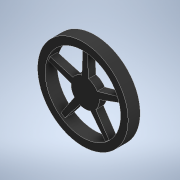
# Autodesk Inventor part: FS90R-W
Saved by Autodesk Inventor 2022 (Build 260153000, 153)
## iProperties
Created: 2024-05-30
Part Number: FS90R-W
Material: 一般
Document SubType Name: Modeling
Designer: yamashita1
Density: 1 g/cm^3
Appearance: ゴム - 黒
Author: yamashita1
Autodesk Inventor part; units mm, degrees
ref_plane "YZ Plane" through (0, 0, 0) normal (1, 0, 0) x (0, 1, 0)
ref_plane "XZ Plane" through (0, 0, 0) normal (0, 1, 0) x (-1, 0, 0)
ref_plane "XY Plane" through (0, 0, 0) normal (0, 0, 1) x (1, 0, 0)
sketch "スケッチ1" plane through (0, 0, 0) normal (0, 0, 1) x (1, 0, 0)
  circle A0 centre (0, 0) radius 30
  circle A1 centre (0, 0) radius 25
  dimension "d0" = 60
  dimension "d1" = 5
  constraints: 2 centre point, 2 coincident
  measures "d0" diameter of A0
  measures "d1" radial gap between concentric circles of A0 A1
extrude "押し出し1" add sketch "スケッチ1" along normal mid plane 8
sketch "スケッチ2" plane through (0, 0, 0) normal (0, 0, 1) x (1, 0, 0)
  circle A0 centre (0, 0) radius 9.35
  line L0 (-1.5, 26) -> (-2.5, 0)
  line L1 (-2.5, 0) -> (2.5, 0)
  line L2 (2.5, 0) -> (1.5, 26)
  line L3 (1.5, 26) -> (-1.5, 26)
  point P0 (0, 26)
  point P1 (-2.15, 9.0994)
  point P2 (2.15, 9.0994)
  dimension "d4" = 18.7
  dimension "d5" = 5
  dimension "d6" = 3
  dimension "d7" = 26
  constraints: 8 end point, 2 coincident, 2 midpoint, 1 centre point, 1 horizontal, 1 parallel, 1 vertical alignment
  measures "d4" diameter of A0
  measures "d5" distance of L0.end L1.end
  measures "d6" distance of L2.end L0.start
  measures "d7" distance between parallel lines of L1 L3
extrude "押し出し2" add sketch "スケッチ2" along normal mid plane 5
pattern_circular "円形状パターン1" count 5 over 360 about axis through (0, 0, -10) along (0, 0, 1) of "押し出し2"
sketch "スケッチ3" plane through (0, 0, -2.5) normal (0, 0, -1) x (-1, 0, 0)
  circle A0 centre (0, 0) radius 3
  dimension "d13" = 6
  constraints: 1 centre point, 1 coincident
  measures "d13" diameter of A0
extrude "押し出し3" add sketch "スケッチ3" along normal blind 3
sketch "スケッチ4" plane through (0, 0, -5.5) normal (0, 0, -1) x (-1, 0, 0)
  circle A0 centre (0, 0) radius 2.43
  dimension "d16" = 4.86
  constraints: 1 centre point, 1 coincident
  measures "d16" diameter of A0
extrude "押し出し4" cut sketch "スケッチ4" against normal blind 3
